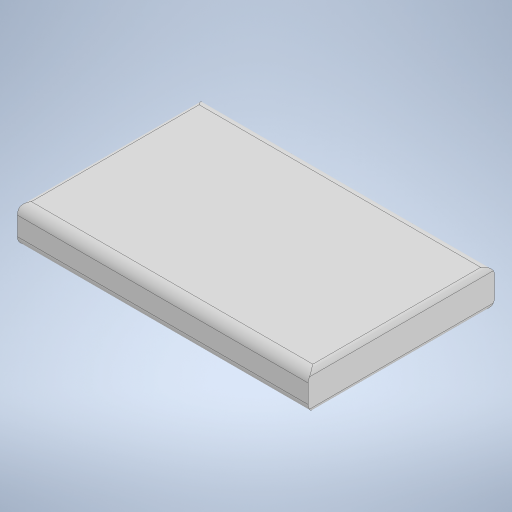
# Autodesk Inventor part: Battery_402030
Saved by Autodesk Inventor 2023 (Build 270158000, 158)
## iProperties
Created: 2023-03-12
Part Number: Battery_402030
Material: Generic
Document SubType Name: Modeling
Designer: nigel
Density: 1 g/cm^3
Appearance: Default
Author: nigel
Autodesk Inventor part; units mm, degrees
ref_plane "YZ Plane" through (0, 0, 0) normal (1, 0, 0) x (0, 1, 0)
ref_plane "XZ Plane" through (0, 0, 0) normal (0, 1, 0) x (-1, 0, 0)
ref_plane "XY Plane" through (0, 0, 0) normal (0, 0, 1) x (1, 0, 0)
sketch "Sketch1" plane through (0, 0, 0) normal (0, 1, 0) x (-1, 0, 0)
  line L0 (15.6, 10) -> (-15.6, 10)
  line L1 (-15.6, 10) -> (-15.6, -10)
  line L2 (-15.6, -10) -> (15.6, -10)
  line L3 (15.6, -10) -> (15.6, 10)
  line L4 (15.6, 10) -> (-15.6, -10) construction
  line L5 (-15.6, 10) -> (15.6, -10) construction
  point P0 (0, 0)
  dimension "d0" = 20
  dimension "d1" = 31.2
  constraints: 12 end point, 2 midpoint, 2 parallel, 1 horizontal, 1 perpendicular
  measures "d0" distance of L0.end L1.end
  measures "d1" distance of L1.end L2.end
extrude "Extrusion1" add sketch "Sketch1" along normal blind 4
fillet "Fillet1" radius 1 4 edges at (0, 4, 10) (0, 0, 10) (0, 4, -10) (0, 0, -10)
fillet "Fillet1" radius 0.5 4 edges at (-15.6, 4, 0) (-15.6, 0, 0) (15.6, 4, 0) (15.6, 0, 0)
body "Solid1"
